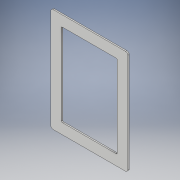
# Autodesk Inventor part: glas-raam
Saved by Autodesk Inventor 2019 (Build 230136000, 136)
## iProperties
Created: 2019-04-26
Part Number: glas-raam
Material: Generic
Document SubType Name: Modeling
Designer: Rene
Density: 1 g/cm^3
Appearance: Default
Author: Rene
Autodesk Inventor part; units mm, degrees
ref_plane "YZ Plane" through (0, 0, 0) normal (1, 0, 0) x (0, 1, 0)
ref_plane "XZ Plane" through (0, 0, 0) normal (0, 1, 0) x (-1, 0, 0)
ref_plane "XY Plane" through (0, 0, 0) normal (0, 0, 1) x (1, 0, 0)
sketch "Sketch1" plane through (0, 0, 0) normal (0, 0, 1) x (1, 0, 0)
  line L0 (165, -222.5) -> (-165, -222.5)
  line L1 (-165, -222.5) -> (-165, 222.5)
  line L2 (-165, 222.5) -> (165, 222.5)
  line L3 (165, 222.5) -> (165, -222.5)
  line L4 (165, -222.5) -> (-165, 222.5) construction
  line L5 (-165, -222.5) -> (165, 222.5) construction
  point P0 (0, 0)
  dimension "d0" = 445
  dimension "d1" = 330
  constraints: 12 end point, 2 midpoint, 2 parallel, 1 horizontal, 1 perpendicular
  measures "d0" distance of L0.end L1.end
  measures "d1" distance of L1.end L2.end
extrude "Extrusion1" add sketch "Sketch1" along normal blind 6
fillet "Fillet1" radius 10 4 edges at (165, 222.5, 3) (-165, 222.5, 3) (165, -222.5, 3) (-165, -222.5, 3)
sketch "Sketch2" plane through (0, 0, 6) normal (0, 0, 1) x (1, 0, 0)
  line L0 (120, -177.5) -> (-120, -177.5)
  line L1 (-120, -177.5) -> (-120, 177.5)
  line L2 (-120, 177.5) -> (120, 177.5)
  line L3 (120, 177.5) -> (120, -177.5)
  line L4 (120, -177.5) -> (-120, 177.5) construction
  line L5 (-120, -177.5) -> (120, 177.5) construction
  point P0 (0, 0)
  dimension "d5" = 355
  dimension "d6" = 240
  constraints: 12 end point, 2 midpoint, 2 parallel, 1 horizontal, 1 perpendicular
  measures "d5" distance of L0.end L1.end
  measures "d6" distance of L0.start L0.end
extrude "Extrusion2" cut sketch "Sketch2" against normal blind 6
fillet "Fillet2" radius 5 4 edges at (-120, 177.5, 3) (120, 177.5, 3) (120, -177.5, 3) (-120, -177.5, 3)
body "Solid1"
